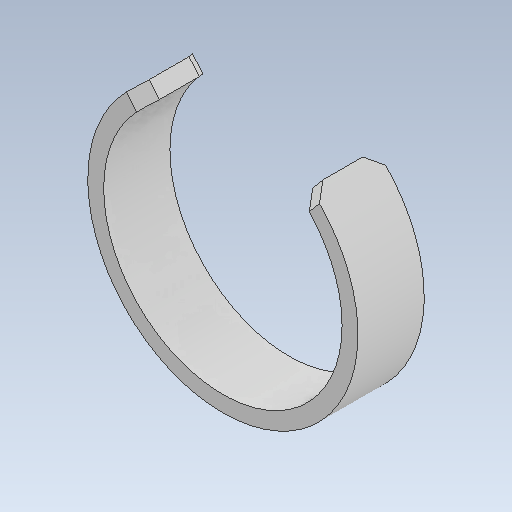
# Autodesk Inventor part: bat_protect_ring
Saved by Autodesk Inventor 2020 (Build 240168000, 168)
## iProperties
Created: 2021-08-28
Part Number: bat_protect_ring
Material: Generic
Document SubType Name: Modeling
Designer: Shuang Peng
Density: 1 g/cm^3
Appearance: Default
Author: Shuang Peng
Autodesk Inventor part; units mm, degrees
ref_plane "YZ Plane" through (0, 0, 0) normal (1, 0, 0) x (0, 1, 0)
ref_plane "XZ Plane" through (0, 0, 0) normal (0, 1, 0) x (-1, 0, 0)
ref_plane "XY Plane" through (0, 0, 0) normal (0, 0, 1) x (1, 0, 0)
sketch "Sketch1" plane through (0, 0, 0) normal (0, 0, 1) x (1, 0, 0)
  circle A0 centre (-8.951, -1.6115) radius 5.2 projected
  circle A1 centre (-8.951, -1.6115) radius 9
  arc A2 (0.6432, -5.0745) -> (1.1277, -0.0431) centre (-8.951, -1.6115) ccw projected
  circle A3 centre (-8.951, -1.6115) radius 10.2
  line L0 (0.049, 8.3885) -> (-1.451, 8.3885) projected
  line L1 (-1.451, 8.3885) -> (-4.951, 8.3885) projected
  arc A4 (-5.4092, 8.0885) -> (-4.951, 8.3885) centre (-5.4092, 8.5885) ccw projected
  line L2 (-5.4092, 8.0885) -> (-12.4927, 8.0885) projected
  arc A5 (-12.951, 8.3885) -> (-12.4927, 8.0885) centre (-12.4927, 8.5885) ccw projected
  line L3 (-12.951, 8.3885) -> (-16.451, 8.3885) projected
  line L4 (-16.451, 8.3885) -> (-17.951, 8.3885) projected
  line L5 (-17.951, 8.3885) -> (-17.951, 2.8885) projected
  line L6 (-17.951, 2.8885) -> (-14.451, 2.8885) projected
  arc A6 (-12.451, 0.8885) -> (-14.451, 2.8885) centre (-14.451, 0.8885) ccw projected
  line L7 (-12.451, 0.8885) -> (-12.451, -6.6115) projected
  line L8 (-12.451, -6.6115) -> (-5.451, -6.6115) projected
  line L9 (-5.451, -6.6115) -> (-5.451, 0.8885) projected
  arc A7 (-3.451, 2.8885) -> (-5.451, 0.8885) centre (-3.451, 0.8885) ccw projected
  line L10 (-3.451, 2.8885) -> (0.049, 2.8885) projected
  line L11 (0.049, 2.8885) -> (0.049, 8.3885) projected
  line L12 (-8.951, -1.6115) -> (-8.951, 8.0885)
  line L13 (-8.951, -1.6115) -> (-2.3946, 6.2021)
  line L14 (-8.951, -1.6115) -> (-15.5074, 6.2021)
  point P0 (0, 0)
  point P1 (-14.7361, 5.2829)
  point P2 (1.1277, -0.0431)
  point P3 (-3.1659, 5.2829)
  dimension "d0" = 18
  dimension "d1" = 20.4
  dimension "d2" = 40
  dimension "d3" = 40
  constraints: 6 end point, 2 centre point, 2 coincident, 2 point on circle, 1 midpoint
  measures "d0" diameter of A1
  measures "d1" diameter of A3
  measures "d2" angle of L12 L13
  measures "d3" angle of L12 L14
extrude "Extrusion1" add sketch "Sketch1" along normal blind 5 contours L13 A3 L11 L10 A1 | L10 L11 A3 A2 L5 L6 A1 | A1 L6 L5 A3 L14
chamfer "Chamfer1" distance 1 angle 45 4 edges at (-15.1217, 5.7425, 5) (-15.1217, 5.7425, 0) (-2.7802, 5.7425, 5) (-2.7802, 5.7425, 0)
body "Solid1"
